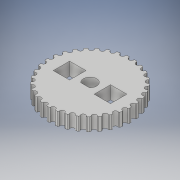
# Autodesk Inventor part: nhk26
Saved by Autodesk Inventor 2019 (Build 230136000, 136)
## iProperties
Created: 2022-02-21
Part Number: nhk26
Material: 一般
Document SubType Name: Modeling
Designer: yuta
Density: 1 g/cm^3
Appearance: 既定
Author: yuta
Autodesk Inventor part; units mm, degrees
ref_plane "YZ Plane" through (0, 0, 0) normal (1, 0, 0) x (0, 1, 0)
ref_plane "XZ Plane" through (0, 0, 0) normal (0, 1, 0) x (-1, 0, 0)
ref_plane "XY Plane" through (0, 0, 0) normal (0, 0, 1) x (1, 0, 0)
sketch "スケッチ1" plane through (0, 0, 0) normal (0, 1, 0) x (-1, 0, 0)
  circle A0 centre (0, 0) radius 26.26 construction
  arc A1 (-1.918, -25.6183) -> (-2.965, -25.5183) centre (0, 0) ccw construction
  circle A2 centre (0, 0) radius 22 construction
  circle A3 centre (0, 0) radius 23.76 construction
  arc A4 (-3.4079, -24.9206) -> (-4.4966, -23.3306) centre (-4.7559, -24.6759) ccw
  arc A5 (0, -23.76) -> (-1.3699, -25.1152) centre (0, -25.13) ccw
  arc A6 (-3.4079, -24.9206) -> (-2.965, -25.5183) centre (-2.9061, -25.0117) ccw
  arc A7 (-1.9388, -25.6163) -> (-1.3699, -25.1152) centre (-1.8799, -25.1097) ccw
  line L0 (0, -23.76) -> (0, 0)
  line L1 (0, 0) -> (-4.4966, -23.3306)
  line L2 (-2.4415, -25.5683) -> (0, 0) construction
  line L3 (-2.965, -25.5183) -> (-2.965, -25.5183)
  arc A8 (-2.965, -25.5183) -> (-1.918, -25.6183) centre (0, 0) ccw
  dimension "d0" = 52.52
  dimension "d1" = 51.38
  dimension "d2" = 44
  dimension "d4" = 47.52
  dimension "d5" = 2.74
  dimension "d6" = 2.74
  dimension "d7" = 1.02
  dimension "d8" = 1.02
  dimension "d10" = 10.909
  dimension "d11" = 5.455
  constraints: 16 point on circle, 9 centre point, 8 end point, 7 tangent, 6 coincident, 1 vertical
  measures "d0" diameter of A0
  measures "d1" diameter of A1
  measures "d2" diameter of A2
  measures "d4" diameter of A3
  measures "d5" diameter of A4
  measures "d6" diameter of A5
  measures "d7" diameter of A6
  measures "d8" diameter of A7
  measures "d10" angle of L1 L0
  measures "d11" angle of L2 L0
extrude "押し出し1" add sketch "スケッチ1" along normal blind 8
pattern_circular "円形状パターン1" count 33 over 360 about axis through (0, 0, 0) along (0, 1, 0) of "押し出し1"
sketch "スケッチ2" plane through (0, 8, 0) normal (0, 1, 0) x (1, 0, 0)
  circle A0 centre (0, 0) radius 4
  line L0 (-17.5, -5) -> (-7.5, -5)
  line L1 (-7.5, -5) -> (-7.5, 5)
  line L2 (-7.5, 5) -> (-17.5, 5)
  line L3 (-17.5, 5) -> (-17.5, -5)
  line L4 (7.5, -5) -> (17.5, -5)
  line L5 (17.5, -5) -> (17.5, 5)
  line L6 (17.5, 5) -> (7.5, 5)
  line L7 (7.5, 5) -> (7.5, -5)
  dimension "d17" = 8
  dimension "d18" = 10
  dimension "d19" = 10
  dimension "d20" = 7.5
  dimension "d21" = 5
  dimension "d22" = 10
  dimension "d23" = 10
  dimension "d24" = 7.5
  constraints: 16 end point, 4 parallel, 2 horizontal, 2 perpendicular, 1 centre point, 1 coincident
  measures "d17" diameter of A0
  measures "d18" distance of L2.end L1.end
  measures "d19" distance of L1.end L0.end
  measures "d20" distance from line of L1 point (0, 0)
  measures "d21" distance from line of point (0, 0) L2
  measures "d22" distance of L6.end L5.end
  measures "d23" distance of L5.end L4.end
  measures "d24" distance from line of L7 point (0, 0)
extrude "押し出し2" cut sketch "スケッチ2" against normal blind 8 contours L3 L2 L1 L0 | L7 L6 L5 L4
sketch "スケッチ3" plane through (0, 8, 0) normal (0, 1, 0) x (1, 0, 0)
  circle A0 centre (0, 0) radius 4
  dimension "d27" = 8
  constraints: 1 centre point, 1 coincident
  measures "d27" diameter of A0
hole "穴1" at (0, 8, 0) direction (0, -1, 0) diameter 8 depth 8
sketch "スケッチ4" plane through (0, 8, 0) normal (0, 1, 0) x (1, 0, 0)
  circle A0 centre (0, 0) radius 4 projected
  line L0 (-2.6458, -3) -> (2.6458, -3)
  point P0 (0, -3)
  dimension "d35" = 3
  constraints: 2 end point, 2 point on circle, 1 horizontal
  measures "d35" distance of point (0, -3) A0.centre
extrude "押し出し3" add sketch "スケッチ4" against normal blind 8 contours L0 A0 picked at (-0.6179, -3.1815)
